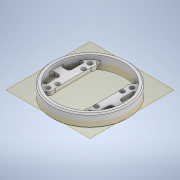
# Autodesk Inventor part: Electro_gps
Saved by Autodesk Inventor 2020 (Build 240168000, 168)
## iProperties
Created: 2020-09-03
Part Number: Electro_gps
Material: Generisch
Document SubType Name: Modeling
Designer: sp
Density: 1 g/cm^3
Appearance: Vorgabe
Author: sp
## iProperties of the stored document _3D-Druck.ipt
Created: 2020-09-03
Part Number: _3D-Druck
Material: Generisch
Document SubType Name: Modeling
Designer: sp
Density: 1 g/cm^3
Appearance: Vorgabe
Author: sp
Autodesk Inventor part; units mm, degrees
ref_plane "YZ Plane" through (0, 0, 0) normal (1, 0, 0) x (0, 1, 0)
ref_plane "XY Plane" through (0, 0, 0) normal (0, 0, 1) x (1, 0, 0)
sketch "Skizze1" plane through (0, 0, 0) normal (0, 1, 0) x (-1, 0, 0)
  circle A0 centre (0, 0) radius 30
  circle A1 centre (0, 0) radius 27
  dimension "d0" = 60
  dimension "d1" = 54
  constraints: 2 centre point, 2 coincident
  measures "d0" diameter of A0
  measures "d1" diameter of A1
extrude "Extrusion1" add sketch "Skizze1" along normal mid plane 10
ref_plane "Arbeitsebene1" through (0, 0, 0) normal (0, 1, 0) x (-1, 0, 0)
chamfer "Fase1" distance 1 angle 45 2 edges at (30, 5, 0) (30, -5, 0)
sketch "Skizze2" plane through (0, 0, 0) normal (0, 1, 0) x (-1, 0, 0)
  line L0 (0, 42.2301) -> (0, -36.7007) construction
  line L1 (32.6355, 0) -> (-32.6355, 0) construction
  line L2 (16.5, 34.419) -> (16.5, -40.3324) construction
  line L3 (-16.5, 35.4304) -> (-16.5, -34.8157) construction
  line L4 (23.5881, 16.5) -> (-32.0387, 16.5) construction
  line L5 (23.5881, -16.5) -> (-39.8541, -16.5) construction
  circle A0 centre (16.5, -16.5) radius 1.75
  circle A1 centre (16.5, 16.5) radius 1.75
  circle A2 centre (-16.5, 16.5) radius 1.75
  circle A3 centre (-16.5, -16.5) radius 1.75
  circle A4 centre (-16.5, 16.5) radius 3.6749
  circle A5 centre (-16.5, -16.5) radius 3.7161
  circle A6 centre (16.5, -16.5) radius 3.7
  circle A7 centre (16.5, 16.5) radius 3.6747
  point P0 (0, 0)
  dimension "d8" = 33
  dimension "d9" = 33
  dimension "d10" = 3.5
  dimension "d11" = 3.5
  dimension "d12" = 3.5
  dimension "d13" = 3.5
  constraints: 12 end point, 9 point on line, 8 centre point, 4 coincident, 3 horizontal, 3 vertical, 1 midpoint, 2 other
  measures "d8" distance between parallel lines of L3 L2
  measures "d9" distance between parallel lines of L4 L5
  measures "d10" diameter of A0
  measures "d11" diameter of A1
  measures "d12" diameter of A2
  measures "d13" diameter of A3
extrude "Extrusion2" add sketch "Skizze2" along normal mid plane 3
fillet "Rundung1" radius 2 16 edges at (-18.7043, 0.75, -19.4718) (-18.7043, -0.75, -19.4718) (-19.4718, 0.75, -18.7043) (-19.4718, -0.75, -18.7043) (-18.8927, 0.75, 19.289) (-18.8927, -0.75, 19.289) (-19.289, 0.75, 18.8927) (-19.289, -0.75, 18.8927) (18.8904, 0.75, 19.2913) (18.8904, -0.75, 19.2913) (19.2913, 0.75, 18.8904) (19.2913, -0.75, 18.8904) (19.551, 0.75, -18.6215) (19.551, -0.75, -18.6215) (18.6215, 0.75, -19.551) (18.6215, -0.75, -19.551)
sketch "Skizze3" plane through (0, 1.5, 0) normal (0, 1, 0) x (1, 0, 0)
  line L0 (-33.5546, 0) -> (36.2487, 0) construction
  line L1 (0, -31.698) -> (0, 37.4161) construction
  circle A0 centre (-15.25, -10.25) radius 1.75
  circle A1 centre (-15.25, 10.25) radius 1.75
  circle A2 centre (15.25, -10.25) radius 1.75
  circle A3 centre (15.25, 10.25) radius 1.75
  line L2 (-15.25, -43.2816) -> (-15.25, 49.413) construction
  line L3 (15.25, -49.7445) -> (15.25, 77.5667) construction
  arc A4 (-14.419, -19.5287) -> (-19.5287, -14.419) centre (-16.5, -16.5) ccw projected
  arc A5 (-19.5455, 14.3988) -> (-22.8871, 14.3241) centre (-21.1918, 13.2631) ccw projected
  line L4 (-13.4713, -14.419) -> (-19.5455, -14.419)
  line L5 (-19.5455, -14.419) -> (-19.5455, 14.3988)
  line L6 (-19.5455, 14.3988) -> (-13.4713, 14.3988)
  line L7 (-13.4713, 14.3988) -> (-13.4713, -14.419)
  arc A6 (19.5289, -14.4189) -> (14.4189, -19.5289) centre (16.5, -16.5) ccw projected
  arc A7 (14.386, 19.5562) -> (19.5562, 14.386) centre (16.5, 16.5) ccw projected
  line L8 (19.565, -14.4724) -> (13.435, -14.4724)
  line L9 (13.435, -14.4724) -> (13.435, 14.3988)
  line L10 (13.435, 14.3988) -> (19.565, 14.3988)
  line L11 (19.565, 14.3988) -> (19.565, -14.4724)
  line L12 (-19.5455, -3.0873) -> (-27, -3.0873)
  line L13 (-27, -3.0873) -> (-27, 3.0873)
  line L14 (-27, 3.0873) -> (-19.5455, 3.0873)
  line L15 (-19.5455, 3.0873) -> (-19.5455, -3.0873)
  line L16 (19.565, -3.0873) -> (27, -3.0873)
  line L17 (27, -3.0873) -> (27, 3.0873)
  line L18 (27, 3.0873) -> (19.565, 3.0873)
  line L19 (19.565, 3.0873) -> (19.565, -3.0873)
  point P0 (0, 0)
  point P1 (18.7479, 13.541)
  point P2 (14.2521, -13.5928)
  dimension "d17" = 3.5
  dimension "d18" = 20.5
  dimension "d19" = 3.5
  dimension "d20" = 20.5
  dimension "d21" = 30.5
  constraints: 40 end point, 9 point on line, 8 parallel, 5 horizontal, 4 centre point, 4 perpendicular, 4 point on circle, 3 vertical, 2 equal radius, 2 symmetric about line, 2 other
  measures "d17" diameter of A1
  measures "d18" distance of A0.centre A1.centre
  measures "d19" diameter of A3
  measures "d20" distance of A2.centre A3.centre
  measures "d21" distance between parallel lines of L3 L2
extrude "Extrusion3" add sketch "Skizze3" against normal blind 3 contours A4 L4 L5 L6 L7 | L12 L13 L14 L5 | L8 L9 L10 L11 | L11 L18 L17 L16
fillet "Rundung2" radius 2 12 edges at (26.8229, 0.75, 3.0873) (26.8229, -0.75, 3.0873) (19.565, 0, 3.0873) (19.565, 0, -3.0873) (26.8229, 0.75, -3.0873) (26.8229, -0.75, -3.0873) (-19.5455, 0, 3.0873) (-26.8229, 0.75, 3.0873) (-26.8229, -0.75, 3.0873) (-26.8229, 0.75, -3.0873) (-26.8229, -0.75, -3.0873) (-19.5455, 0, -3.0873)
fillet "Rundung3" radius 2 8 edges at (-13.4713, 0.75, -14.3746) (-13.4713, -0.75, -14.3746) (-13.4713, -0.75, 14.419) (-13.4713, 0.75, 14.419) (13.435, 0.75, 14.4724) (13.435, -0.75, 14.4724) (13.435, 0.75, -14.3988) (13.435, -0.75, -14.3988)
